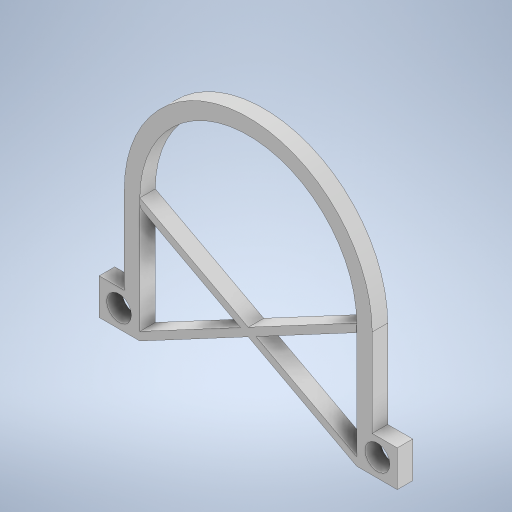
# Autodesk Inventor part: łapka
Saved by Autodesk Inventor 2023 (Build 270158000, 158)
## iProperties
Created: 2023-02-09
Part Number: łapka
Material: Ogólny
Document SubType Name: Modeling
Designer: User
Density: 1 g/cm^3
Appearance: Domyślna
Author: User
Autodesk Inventor part; units mm, degrees
ref_plane "YZ Plane" through (0, 0, 0) normal (1, 0, 0) x (0, 1, 0)
ref_plane "XZ Plane" through (0, 0, 0) normal (0, 1, 0) x (-1, 0, 0)
ref_plane "XY Plane" through (0, 0, 0) normal (0, 0, 1) x (1, 0, 0)
sketch "Szkic1" plane through (0, 0, 0) normal (0, 0, 1) x (1, 0, 0)
  circle A0 centre (0, 0) radius 20
  circle A1 centre (0, 0) radius 17.5
  line L0 (-20, 0) -> (-17.5, 0)
  line L1 (-17.5, 0) -> (-17.5, -20)
  line L2 (-17.5, -20) -> (-20, -20)
  line L3 (-20, -20) -> (-20, 0)
  line L4 (17.5, 0) -> (20, 0)
  line L5 (20, 0) -> (20, -20)
  line L6 (20, -20) -> (17.5, -20)
  line L7 (17.5, -20) -> (17.5, 0)
  line L8 (-20, 0) -> (17.5, -20)
  line L9 (-17.5, 0) -> (20, -20)
  line L10 (-20, -20) -> (17.5, 0)
  line L11 (-17.5, -20) -> (20, 0)
  line L12 (17.5, -20) -> (24.0492, -20)
  line L13 (24.0492, -20) -> (24.0492, -14.1676)
  line L14 (24.0492, -14.1676) -> (17.5, -14.1676)
  line L15 (17.5, -14.1676) -> (17.5, -20)
  line L16 (0, 24.8305) -> (0, -32.2355)
  line L17 (-17.5, -20) -> (-24.0492, -20)
  line L18 (-24.0492, -20) -> (-24.0492, -14.1676)
  line L19 (-24.0492, -14.1676) -> (-17.5, -14.1676)
  line L20 (-17.5, -14.1676) -> (-17.5, -20)
  circle A2 centre (20.7746, -17.0838) radius 2.2775
  circle A3 centre (-20.7746, -17.0838) radius 2.2775
  point P0 (17.5, -18.6667)
  point P1 (1.25, -10)
  point P2 (17.4469, -1.3616)
  point P3 (0, -9.3333)
  point P4 (-17.4469, -1.3616)
  point P5 (-1.25, -10)
  point P6 (-17.5, -18.6667)
  point P7 (0, -10.6667)
  point P8 (-20, -14.1676)
  point P9 (20, -14.1676)
  dimension "d1" = 35
  dimension "d0" = 40
  dimension "d2" = 20
  dimension "d3" = 2.5
  dimension "d4" = 2.5
  dimension "d5" = 20
  constraints: 42 end point, 6 parallel, 4 symmetric about line, 3 centre point, 3 horizontal, 3 perpendicular, 2 coincident, 2 point on circle, 1 point on line, 1 vertical, 4 other
  measures "d0" diameter of A0
  measures "d2" distance between parallel lines of L2 L0
  measures "d3" distance of L0.start L0.end
  measures "d4" distance of L4.start L4.end
  measures "d5" distance of L4.end L5.end
extrude "Wyciągnięcie proste3" add sketch "Szkic1" along normal blind 2.5 contours L4 A1 L16 A0 | L5 L14 L7 A0 | L11 L7 L4 | A0 L7 L11 | L16 A1 L0 A0 | A1 L11 L9 L10 | L14 L13 L12 L5 A2 | L5 A2 L9 L7 L14 | L8 L1 A0 | A0 L1 L19 L3 | L0 L1 L8 | L9 L7 L8 A0 | A0 L8 A1 L9 | L10 L8 A1 L9 | L16 L8 L10 | L9 L11 L16 | A2 L5 | L5 A2 | L19 L1 L10 L3 A3 | L3 A3 L17 L18 L19 | A1 L8 L11 L9 | L9 L6 L7 | L8 L11 A1 L10 | L10 A1 L11 A0 | A0 L11 L1 L10 | A3 L3 | L3 A3 | L1 L2 L10
sketch "Szkic2" plane through (0, 0, 0) normal (0, 0, -1) x (-1, 0, 0)
  circle A0 centre (-20.8556, -17.0848) radius 2.22
  line L0 (0, 8.6255) -> (0, -29.7985)
  circle A1 centre (20.8556, -17.0848) radius 2.22
  point P0 (0, 0)
  dimension "d14" = 4.4401
  constraints: 2 centre point, 2 end point, 1 symmetric about line, 1 vertical, 1 other
  measures "d14" diameter of A0
hole "Otwór1" at (20.8556, -17.0848, 0) at (-20.8556, -17.0848, 0) direction (0, 0, 1) diameter 4 end through all
